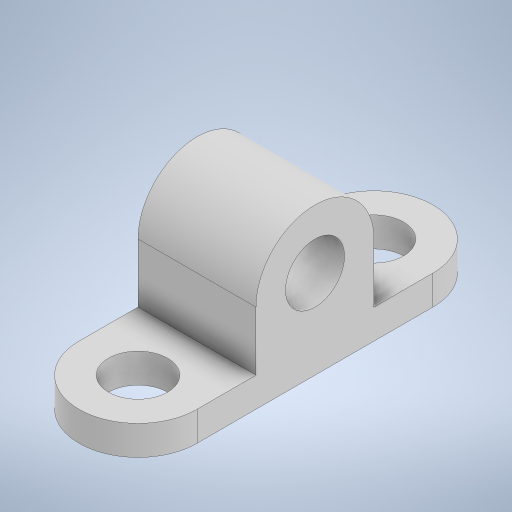
# Autodesk Inventor part: Tarea 1 - Dinámica
Saved by Autodesk Inventor 2023 (Build 270158000, 158)
## iProperties
Created: 2024-01-31
Part Number: Tarea 1 - Dinámica
Material: Genérico
Document SubType Name: Modeling
Designer: karen
Density: 1 g/cm^3
Appearance: Valor por defecto
Author: karen
Autodesk Inventor part; units mm, degrees
ref_plane "YZ Plane" through (0, 0, 0) normal (1, 0, 0) x (0, 1, 0)
ref_plane "XZ Plane" through (0, 0, 0) normal (0, 1, 0) x (-1, 0, 0)
ref_plane "XY Plane" through (0, 0, 0) normal (0, 0, 1) x (1, 0, 0)
sketch "Boceto1" plane through (0, 0, 0) normal (0, 1, 0) x (-1, 0, 0)
  line L0 (20, 20) -> (20, -20)
  line L1 (-20, -20) -> (-20, 20)
  line L2 (20, 20) -> (-20, -20) construction
  line L3 (20, -20) -> (-20, 20) construction
  line L4 (0, 20) -> (0, 40) construction
  line L5 (0, -20) -> (0, -40) construction
  circle A0 centre (0, 40) radius 10
  arc A1 (20, 40) -> (-20, 40) centre (0, 40) ccw
  circle A2 centre (0, -40) radius 10
  arc A3 (-20, -40) -> (20, -40) centre (0, -40) ccw
  line L6 (20, 40) -> (20, 20)
  line L7 (-20, 40) -> (-20, 20)
  line L8 (-20, -20) -> (-20, -40)
  line L9 (20, -20) -> (20, -40)
  arc A4 (20, 40) -> (-20, 40) centre (0, 40) ccw
  point P0 (0, 0)
  dimension "d8" = 20
  dimension "d9" = 20
  dimension "d10" = 40
  dimension "d11" = 40
  dimension "d12" = 40
  dimension "d13" = 40
  constraints: 20 end point, 6 point on circle, 5 centre point, 5 coincident, 3 point on line, 3 vertical, 2 midpoint, 2 parallel
  measures "d8" diameter of A0
  measures "d9" diameter of A2
  measures "d10" diameter of A3
  measures "d11" diameter of A4
  measures "d12" distance from line of L0 L1.start
  measures "d13" distance of L1.start L1.end
extrude "Extrusión1" add sketch "Boceto1" along normal blind 10
sketch "Boceto2" plane through (20, 0, 40) normal (1, 0, 0) x (0, 0, -1)
  line L0 (0, 10) -> (80, 10) construction
  line L1 (40, 10) -> (40, 30) construction
  arc A0 (60, 30) -> (20, 30) centre (40, 30) ccw
  circle A1 centre (40, 30) radius 10
  line L2 (20, 30) -> (20, 10)
  line L3 (60, 30) -> (60, 10)
  line L4 (20, 10) -> (60, 10)
  point P0 (40, 0)
  dimension "d19" = 20
  constraints: 8 end point, 2 centre point, 2 coincident, 2 midpoint, 2 perpendicular, 2 point on circle, 2 point on line, 1 collinear, 1 vertical
  measures "d19" diameter of A1
extrude "Extrusión2" add sketch "Boceto2" against normal blind 40
